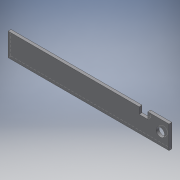
# Autodesk Inventor part: Spoiler
Saved by Autodesk Inventor 2019 (Build 230136000, 136)
## iProperties
Created: 2018-11-27
Part Number: Spoiler
Material: Generic
Document SubType Name: Modeling
Designer: Andres
Density: 1 g/cm^3
Appearance: Default
Author: Andres
Autodesk Inventor part; units mm, degrees
ref_plane "YZ Plane" through (0, 0, 0) normal (1, 0, 0) x (0, 1, 0)
ref_plane "XZ Plane" through (0, 0, 0) normal (0, 1, 0) x (-1, 0, 0)
ref_plane "XY Plane" through (0, 0, 0) normal (0, 0, 1) x (1, 0, 0)
sketch "Sketch1" plane through (0, 0, 0) normal (0, 0, 1) x (1, 0, 0)
  line L0 (3, -4) -> (-53, -4)
  line L1 (-53, -4) -> (-53, 4)
  line L2 (-53, 4) -> (3, 4)
  line L3 (3, 4) -> (3, -4)
  circle A0 centre (0, 0) radius 1.5 projected
  point P0 (0, 0)
  point P1 (-53, 3)
  dimension "d0" = 8
  dimension "d1" = 56
  dimension "d2" = 4
  constraints: 8 end point, 2 parallel, 1 horizontal, 1 perpendicular, 1 other
  measures "d0" distance of L0.end L1.end
  measures "d1" distance of L0.start L0.end
  measures "d2" distance from line of L0 point (0, 0)
extrude "Extrusion2" add sketch "Sketch1" along normal blind 1
sketch "Sketch2" plane through (0, 0, 1) normal (0, 0, 1) x (1, 0, 0)
  line L0 (-4.4, 1.7167) -> (-7.7768, 1.7167)
  line L1 (-7.7768, 1.7167) -> (-7.7768, 4)
  line L2 (3, 4) -> (-53, 4) projected
  line L3 (-4.4, 4) -> (-7.7768, 4)
  line L4 (-4.4, 1.7167) -> (-4.1, 1.7167)
  line L5 (-4.1, 1.7167) -> (-4.1, 4)
  line L6 (-4.1, 4) -> (-4.4, 4)
  point P0 (0, 0)
  dimension "d10" = 0.3
  constraints: 12 end point, 3 point on line, 2 perpendicular, 1 collinear, 1 horizontal
  measures "d10" distance of L0.start L4.end
extrude "Extrusion3" cut sketch "Sketch2" against normal blind 10
body "Solid2"
